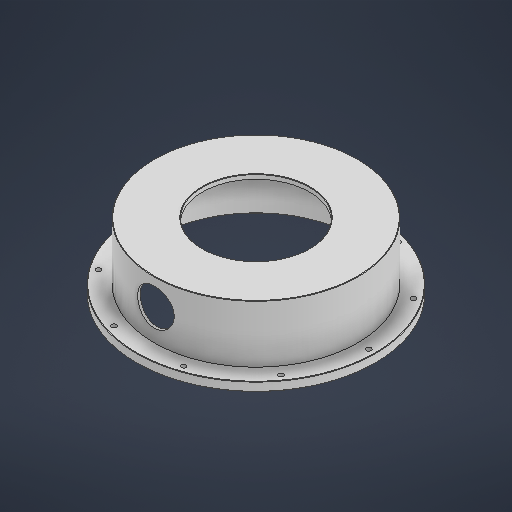
# Autodesk Inventor part: Cylinder  Segment - 01
Saved by Autodesk Inventor 2025 (Build 290162000, 162)
## iProperties
Created: 2024-04-11
Part Number: Cylinder  Segment - 01
Material: Generic
Document SubType Name: Modeling
Designer: Thienan Hoang
Density: 1 g/cm^3
Appearance: Default
Author: Thienan Hoang
Autodesk Inventor part; units mm, degrees
ref_plane "YZ Plane" through (0, 0, 0) normal (1, 0, 0) x (0, 1, 0)
ref_plane "XZ Plane" through (0, 0, 0) normal (0, 1, 0) x (-1, 0, 0)
ref_plane "XY Plane" through (0, 0, 0) normal (0, 0, 1) x (1, 0, 0)
sketch "Sketch1" plane through (0, 0, 0) normal (0, 1, 0) x (-1, 0, 0)
  circle A0 centre (0, 0) radius 135
  circle A1 centre (0, 0) radius 115
  circle A2 centre (0, 0) radius 112.0375
  circle A3 centre (0, 0) radius 9.5
  dimension "Absolute_Diameter" = 270
  dimension "Diameter_No_Outer_Lip" = 230
  dimension "Inner_Cylinder_Diameter" = 224.075
  dimension "Lip_Diameter" = 19
  constraints: 4 centre point, 4 coincident
  measures "Absolute_Diameter" diameter of A0
  measures "Diameter_No_Outer_Lip" diameter of A1
  measures "Inner_Cylinder_Diameter" diameter of A2
  measures "Lip_Diameter" diameter of A3
extrude "Extrusion1" add sketch "Sketch1" along normal blind 10 contours A0
extrude "Extrusion2" add sketch "Sketch1" along normal blind 75 contours A1
sketch "Sketch2" plane through (0, 75, 0) normal (0, 1, 0) x (1, 0, 0)
  circle A0 centre (0, 0) radius 115
  circle A1 centre (0, 0) radius 60.375
  dimension "Lip_Diameter_Out" = 230
  dimension "Inner_Lip_Diameter" = 120.75
  constraints: 2 centre point, 1 coincident
  measures "Lip_Diameter_Out" diameter of A0
  measures "Inner_Lip_Diameter" diameter of A1
extrude "Extrusion7" add sketch "Sketch2" against normal blind 5
chamfer "Chamfer1" distance 0.5 angle 45 2 edges at (115, 75, 0) (-60.375, 75, 0)
chamfer "Chamfer2" distance 0.5 angle 45 3 edges at (135, 10, 0) (135, 0, 0) (112.0375, 0, 0)
sketch "Sketch3" plane through (0, 10, 0) normal (0, 1, 0) x (1, 0, 0)
  circle A0 centre (0, 0) radius 127.5
  circle A1 centre (-127.5, 0) radius 2.75
  circle A2 centre (-103.1497, -74.9426) radius 2.75
  circle A3 centre (-39.3997, -121.2597) radius 2.75
  circle A4 centre (39.3997, -121.2597) radius 2.75
  circle A5 centre (103.1497, -74.9426) radius 2.75
  circle A6 centre (127.5, 0) radius 2.75
  circle A7 centre (103.1497, 74.9426) radius 2.75
  circle A8 centre (39.3997, 121.2597) radius 2.75
  circle A9 centre (-39.3997, 121.2597) radius 2.75
  circle A10 centre (-103.1497, 74.9426) radius 2.75
  dimension "d27" = 255
  dimension "d28" = 5.5
  dimension "d31" = 360
  constraints: 10 centre point, 1 coincident, 1 horizontal alignment, 23 other
  measures "d28" diameter of A1
extrude "Extrusion8" cut sketch "Sketch3" against normal blind 10 contours A0 A6 | A0 A6 | A7 A0 | A0 A7 | A5 A0 | A0 A5 | A8 A0 | A0 A8 | A4 A0 | A0 A4 | A9 A0 | A0 A9 | A3 A0 | A0 A3 | A10 A0 | A0 A10 | A2 A0 | A0 A2 | A1 A0 | A0 A1
chamfer "Chamfer3" [suppressed]
sketch "Sketch5" plane through (0, 75, 0) normal (0, 1, 0) x (1, 0, 0)
  circle A0 centre (0, 0) radius 39.5
  circle A1 centre (0, 0) radius 112.5375 projected
  line L0 (105.9252, 8.8939) -> (105.9252, -41.1061)
  line L1 (-117.4998, -25) -> (-117.4998, 25)
  line L2 (-117.4998, 25) -> (-51.7808, 25)
  line L3 (56.808, 8.8939) -> (105.9252, 8.8939)
  line L4 (105.9252, -41.1061) -> (40.2062, -41.1061)
  line L5 (-51.7808, -25) -> (-117.4998, -25)
  arc A2 (-51.7808, -25) -> (40.2062, -41.1061) centre (0, 0) ccw
  arc A3 (56.808, 8.8939) -> (-51.7808, 25) centre (0, 0) ccw
  dimension "d54" = 50
  dimension "d97" = 65.719
  dimension "d98" = 65.719
  dimension "d99" = 57.5
  dimension "d100" = 57.5
  dimension "d101" = 50
  dimension "d102" = 50
  dimension "d103" = 52.6842
  dimension "d104" = 223.425
  constraints: 12 end point, 5 parallel, 4 point on circle, 3 centre point, 2 coincident, 2 horizontal, 2 perpendicular
  measures "d54" distance of L0.start L0.end
  measures "d97" distance of L5.start L1.start
  measures "d98" distance of L0.end L4.end
  measures "d99" radius of A2
  measures "d100" radius of A3
  measures "d101" distance of L1.start L1.end
  measures "d102" distance of L5.start L2.end
  measures "d103" distance of L4.end L3.start
  measures "d104" distance between parallel lines of L0 L1
extrude "Extrusion9" [suppressed]
sketch "Sketch6" plane through (0, 75, 0) normal (0, -1, 0) x (1, 0, 0)
  line L0 (111.7125, -22) -> (-111.7125, -22)
  line L1 (-111.7125, -22) -> (-111.7125, 22)
  line L2 (-111.7125, 22) -> (111.7125, 22)
  line L3 (111.7125, 22) -> (111.7125, -22)
  line L4 (111.7125, -22) -> (-111.7125, 22) construction
  line L5 (-111.7125, -22) -> (111.7125, 22) construction
  line L6 (139.9625, -19.625) -> (86.4625, -19.625)
  line L7 (83.4625, -16.625) -> (83.4625, 16.625)
  line L8 (86.4625, 19.625) -> (139.9625, 19.625)
  line L9 (139.9625, 19.625) -> (139.9625, -19.625)
  line L10 (139.9625, -19.625) -> (83.4625, 19.625) construction
  line L11 (83.4625, -19.625) -> (139.9625, 19.625) construction
  line L12 (-86.4625, -19.625) -> (-139.9625, -19.625)
  line L13 (-139.9625, -19.625) -> (-139.9625, 19.625)
  line L14 (-139.9625, 19.625) -> (-86.4625, 19.625)
  line L15 (-83.4625, 16.625) -> (-83.4625, -16.625)
  line L16 (-83.4625, -19.625) -> (-139.9625, 19.625) construction
  line L17 (-139.9625, -19.625) -> (-83.4625, 19.625) construction
  arc A0 (-86.4625, -19.625) -> (-83.4625, -16.625) centre (-86.4625, -16.625) ccw
  arc A1 (-83.4625, 16.625) -> (-86.4625, 19.625) centre (-86.4625, 16.625) ccw
  arc A2 (83.4625, -16.625) -> (86.4625, -19.625) centre (86.4625, -16.625) ccw
  arc A3 (86.4625, 19.625) -> (83.4625, 16.625) centre (86.4625, 16.625) ccw
  point P0 (0, 0)
  point P1 (111.7125, 0)
  point P2 (-111.7125, 0)
  dimension "d58" = 234.5
  dimension "d59" = 44
  dimension "d60" = 56.5
  dimension "d61" = 39.25
  dimension "d62" = 56.5
  dimension "d63" = 39.25
  dimension "d64" = 3
  constraints: 36 end point, 8 midpoint, 8 point on circle, 8 point on line, 8 tangent, 6 parallel, 4 centre point, 3 equal radius, 3 horizontal, 3 perpendicular
  measures "d59" distance of L0.end L1.end
  measures "d60" distance of L10.end L8.end
  measures "d61" distance of L11.start L10.end
  measures "d62" distance of L13.end L17.end
  measures "d63" distance of L12.end L13.end
  measures "d64" radius of A0
extrude "Extrusion10" [suppressed]
sketch "Sketch8" plane through (0, 95, 0) normal (0, 1, 0) x (1, 0, 0)
  line L0 (-92.7125, 11) -> (92.7125, 11)
  line L1 (92.7125, 11) -> (92.7125, -11)
  line L2 (92.7125, -11) -> (-92.7125, -11)
  line L3 (-92.7125, -11) -> (-92.7125, 11)
  line L4 (-92.7125, 11) -> (92.7125, -11) construction
  line L5 (92.7125, 11) -> (-92.7125, -11) construction
  circle A0 centre (-92.7125, 11) radius 3.75
  circle A1 centre (-92.7125, -11) radius 3.75
  circle A2 centre (92.7125, 11) radius 3.75
  circle A3 centre (92.7125, -11) radius 3.75
  point P0 (0, 0)
  dimension "d69" = 197
  dimension "d70" = 6.35
  dimension "d71" = 4.5
  dimension "d72" = 7.5
  dimension "d73" = 7.5
  dimension "d74" = 7.5
  constraints: 12 end point, 4 centre point, 4 coincident, 2 midpoint, 2 parallel, 1 horizontal, 1 perpendicular
  measures "d72" diameter of A1
  measures "d73" diameter of A2
  measures "d74" diameter of A3
hole "Hole2" [suppressed]
hole "Hole3" [suppressed]
chamfer "Chamfer4" [suppressed]
fillet "Fillet1" [suppressed]
fillet "Fillet2" [suppressed]
chamfer "Chamfer5" [suppressed]
sketch "Sketch9" plane through (0, 95, 0) normal (0, 1, 0) x (1, 0, 0)
  line L0 (-68.2625, 6.35) -> (-65.0875, 6.35)
  line L1 (-65.0875, 6.35) -> (-65.0875, -6.35)
  line L2 (-65.0875, -6.35) -> (-68.2625, -6.35)
  line L3 (-68.2625, -6.35) -> (-68.2625, 6.35)
  line L4 (-68.2625, 6.35) -> (-65.0875, -6.35) construction
  line L5 (-65.0875, 6.35) -> (-68.2625, -6.35) construction
  line L6 (-68.2625, -6.35) -> (-66.675, -10.3402)
  line L7 (-66.675, -10.3402) -> (-65.0875, -6.35)
  point P0 (0, 0)
  point P1 (-66.675, 0)
  constraints: 16 end point, 2 midpoint, 2 parallel, 1 horizontal, 1 perpendicular
extrude "Extrusion11" [suppressed]
sketch "Sketch12" plane through (0, 75, 0) normal (0, 1, 0) x (1, 0, 0)
  circle A0 centre (0, 0) radius 40
  circle A1 centre (40, 0) radius 1.25
  circle A2 centre (20, 34.641) radius 1.25
  circle A3 centre (-20, 34.641) radius 1.25
  circle A4 centre (-40, 0) radius 1.25
  circle A5 centre (-20, -34.641) radius 1.25
  circle A6 centre (20, -34.641) radius 1.25
  dimension "d115" = 80
  dimension "d116" = 2.5
  dimension "d119" = 360
  constraints: 6 centre point, 1 coincident, 1 horizontal alignment, 15 other
  measures "d116" diameter of A1
hole "Hole4" [suppressed]
sketch "Sketch13" plane through (0, 0, 0) normal (0, 0, 1) x (1, 0, 0)
  circle A0 centre (0, 45) radius 20.625
  line L0 (134.5, 0) -> (-134.5, 0) projected
  point P0 (0, 0)
  dimension "d128" = 41.25
  dimension "d129" = 45
  constraints: 1 centre point
  measures "d128" diameter of A0
  measures "d129" distance from line of L0 A0.centre
extrude "Extrusion14" cut sketch "Sketch13" along normal through all
body "Solid1"
